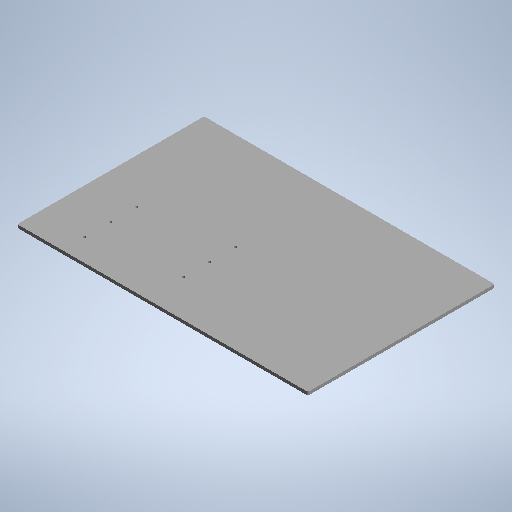
# Autodesk Inventor part: TB_FRM_MC_001_BasePlate
Saved by Autodesk Inventor 2025.4 (Build 294407000, 407)
## iProperties
Created: 2026-06-26
Part Number: TB_FRM_MC_001_BasePlate
Material: Générique
Document SubType Name: Modeling
Designer: louis
Density: 1 g/cm^3
Appearance: Par défaut
Author: louis
Autodesk Inventor part; units mm, degrees
ref_plane "YZ Plane" through (0, 0, 0) normal (1, 0, 0) x (0, 1, 0)
ref_plane "XZ Plane" through (0, 0, 0) normal (0, 1, 0) x (-1, 0, 0)
ref_plane "XY Plane" through (0, 0, 0) normal (0, 0, 1) x (1, 0, 0)
sketch "Sketch2" plane through (0, 0, 0) normal (0, 0, 1) x (1, 0, 0)
  line L0 (278.5, 179) -> (-278.5, 179)
  line L1 (-278.5, 179) -> (-278.5, -179)
  line L2 (-278.5, -179) -> (278.5, -179)
  line L3 (278.5, -179) -> (278.5, 179)
  line L4 (278.5, 179) -> (-278.5, -179) construction
  line L5 (-278.5, 179) -> (278.5, -179) construction
  point P0 (0, 0)
  dimension "d0" = 557
  dimension "d1" = 358
  constraints: 12 end point, 2 midpoint, 2 parallel, 1 horizontal, 1 perpendicular
  measures "d0" distance of L2.end L1.end
  measures "d1" distance of L0.end L1.end
extrude "Extrusion1" add sketch "Sketch2" against normal blind 6
fillet "Fillet1" radius 3 4 edges at (-278.5, -179, -3) (-278.5, 179, -3) (278.5, -179, -3) (278.5, 179, -3)
sketch "Sketch3" plane through (0, 0, 0) normal (0, 0, 1) x (1, 0, 0)
  line L0 (-192.9588, -135.4581) -> (-192.9588, -85.4581) construction
  line L1 (-192.9588, -85.4581) -> (-192.9588, -35.4581) construction
  line L2 (-192.9588, -135.4581) -> (-31.9588, -107.4581) construction
  line L3 (-192.9588, -85.4581) -> (-31.9588, -57.4581) construction
  line L4 (-192.9588, -35.4581) -> (-31.9588, -7.4581) construction
  line L5 (-197.4588, -141.4581) -> (-27.4588, -141.4581)
  line L6 (-27.4588, -141.4581) -> (-27.4588, -101.4581)
  line L7 (-27.4588, -101.4581) -> (-197.4588, -101.4581)
  line L8 (-197.4588, -101.4581) -> (-197.4588, -141.4581)
  line L9 (-197.4588, -141.4581) -> (-27.4588, -101.4581) construction
  line L10 (-27.4588, -141.4581) -> (-197.4588, -101.4581) construction
  line L11 (-197.4588, -91.4581) -> (-27.4588, -91.4581)
  line L12 (-27.4588, -91.4581) -> (-27.4588, -51.4581)
  line L13 (-27.4588, -51.4581) -> (-197.4588, -51.4581)
  line L14 (-197.4588, -51.4581) -> (-197.4588, -91.4581)
  line L15 (-197.4588, -91.4581) -> (-27.4588, -51.4581) construction
  line L16 (-27.4588, -91.4581) -> (-197.4588, -51.4581) construction
  line L17 (-197.4588, -41.4581) -> (-27.4588, -41.4581)
  line L18 (-27.4588, -41.4581) -> (-27.4588, -1.4581)
  line L19 (-27.4588, -1.4581) -> (-197.4588, -1.4581)
  line L20 (-197.4588, -1.4581) -> (-197.4588, -41.4581)
  line L21 (-197.4588, -41.4581) -> (-27.4588, -1.4581) construction
  line L22 (-27.4588, -41.4581) -> (-197.4588, -1.4581) construction
  line L23 (22.5412, -161.4581) -> (-247.4588, -161.4581)
  line L24 (-247.4588, -161.4581) -> (-247.4588, 18.5419)
  line L25 (-247.4588, 18.5419) -> (22.5412, 18.5419)
  line L26 (22.5412, 18.5419) -> (22.5412, -161.4581)
  line L27 (22.5412, -161.4581) -> (-247.4588, 18.5419) construction
  line L28 (-247.4588, -161.4581) -> (22.5412, 18.5419) construction
  point P0 (0, 0)
  point P1 (-112.4588, -121.4581)
  point P2 (-112.4588, -71.4581)
  point P3 (-112.4588, -21.4581)
  dimension "d12" = 28
  dimension "d13" = 161
  dimension "d14" = 161
  dimension "d15" = 28
  dimension "d16" = 28
  dimension "d17" = 161
  dimension "d18" = 50
  dimension "d19" = 50
  dimension "d20" = 170
  dimension "d21" = 40
  dimension "d22" = 170
  dimension "d23" = 40
  dimension "d24" = 170
  dimension "d25" = 40
  dimension "d26" = 20
  dimension "d27" = 50
  constraints: 58 end point, 11 midpoint, 8 parallel, 4 horizontal, 4 perpendicular, 2 vertical
  measures "d12" vertical distance of L2.end L0.start
  measures "d13" horizontal distance of L0.start L2.end
  measures "d14" horizontal distance of L3.end L0.end
  measures "d15" vertical distance of L3.end L0.end
  measures "d16" vertical distance of L4.end L1.end
  measures "d17" horizontal distance of L4.end L1.end
  measures "d18" distance of L0.start L0.end
  measures "d19" distance of L0.end L1.end
  measures "d20" distance of L7.end L6.end
  measures "d21" distance of L6.end L5.end
  measures "d22" distance of L13.end L12.end
  measures "d23" distance of L12.end L11.end
  measures "d24" distance of L19.end L18.end
  measures "d25" distance of L18.end L17.end
  measures "d26" distance between parallel lines of L25 L19
  measures "d27" distance between parallel lines of L14 L24
hole "Hole1" at (-192.9588, -135.4581, 0) at (-31.9588, -107.4581, 0) at (-192.9588, -85.4581, 0) at (-31.9588, -7.4581, 0) at (-31.9588, -57.4581, 0) at (-192.9588, -35.4581, 0) direction (0, 0, -1) diameter 4.5 end through all clearance for "Flat Head Machine Screw" size "M4" standard "Ansi Metric M Profile"
body "Solid1"
